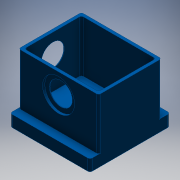
# Autodesk Inventor part: sampleChamber_singlePiece_filipeSample
Saved by Autodesk Inventor 2016 (Build 200138000, 138)
## iProperties
Created: 2016-04-10
Part Number: sampleChamber_singlePiece_filipeSample
Material: Generic
Document SubType Name: Modeling
Designer: sims01
Density: 1 g/cm^3
Appearance: Default
Author: sims01
Autodesk Inventor part; units mm, degrees
ref_plane "YZ Plane" through (0, 0, 0) normal (1, 0, 0) x (0, 1, 0)
ref_plane "XZ Plane" through (0, 0, 0) normal (0, 1, 0) x (-1, 0, 0)
ref_plane "XY Plane" through (0, 0, 0) normal (0, 0, 1) x (1, 0, 0)
sketch "Sketch1" plane through (0, 0, 0) normal (0, 0, 1) x (1, 0, 0)
  line L0 (-33, 35) -> (33, 35)
  line L1 (35, 33) -> (35, -33)
  line L2 (33, -35) -> (-33, -35)
  line L3 (-35, -33) -> (-35, 33)
  arc A0 (-35, -33) -> (-33, -35) centre (-33, -33) ccw
  arc A1 (-33, 35) -> (-35, 33) centre (-33, 33) ccw
  arc A2 (35, 33) -> (33, 35) centre (33, 33) ccw
  arc A3 (33, -35) -> (35, -33) centre (33, -33) ccw
  point P0 (0, 0)
  point P1 (-35, 35)
  point P2 (35, -35)
  point P3 (35, 35)
  point P4 (-35, -35)
  dimension "d0" = 70
  dimension "d1" = 35
  dimension "d2" = 70
  dimension "d3" = 35
  dimension "d85" = 2
  constraints: 8 end point, 8 point on circle, 8 point on line, 8 tangent, 4 centre point, 3 equal radius, 2 parallel, 1 horizontal, 1 perpendicular
  measures "d0" distance of point (35, -35) point (-35, -35)
  measures "d1" distance from line of point (0, 0) L1
  measures "d2" distance of point (-35, -35) point (-35, 35)
  measures "d3" distance from line of point (0, 0) L0
  measures "d85" radius of A0
extrude "Extrusion1" add sketch "Sketch1" along normal blind 10
sketch "Sketch3" plane through (0, 0, 10) normal (0, 0, 1) x (1, 0, 0)
  line L0 (-33, 27.5) -> (33, 27.5)
  line L1 (35, 25.5) -> (35, -25.5)
  line L2 (33, -27.5) -> (-33, -27.5)
  line L3 (-35, -25.5) -> (-35, 25.5)
  line L4 (-35, 33) -> (-35, -33) projected
  line L5 (-30.5, 25) -> (30.5, 25)
  line L6 (32.5, 23) -> (32.5, -23)
  line L7 (30.5, -25) -> (-30.5, -25)
  line L8 (-32.5, -23) -> (-32.5, 23)
  arc A0 (-35, -25.5) -> (-33, -27.5) centre (-33, -25.5) ccw
  arc A1 (-32.5, -23) -> (-30.5, -25) centre (-30.5, -23) ccw
  arc A2 (33, -27.5) -> (35, -25.5) centre (33, -25.5) ccw
  arc A3 (30.5, -25) -> (32.5, -23) centre (30.5, -23) ccw
  arc A4 (32.5, 23) -> (30.5, 25) centre (30.5, 23) ccw
  arc A5 (-30.5, 25) -> (-32.5, 23) centre (-30.5, 23) ccw
  arc A6 (-33, 27.5) -> (-35, 25.5) centre (-33, 25.5) ccw
  arc A7 (35, 25.5) -> (33, 27.5) centre (33, 25.5) ccw
  point P0 (0, 0)
  point P1 (-35, 27.5)
  point P2 (35, -27.5)
  point P3 (35, 27.5)
  point P4 (-35, -27.5)
  point P5 (-35, 35)
  point P6 (-35, -35)
  point P7 (-32.5, 25)
  point P8 (32.5, -25)
  point P9 (32.5, 25)
  point P10 (-32.5, -25)
  dimension "d17" = 70
  dimension "d18" = 55
  dimension "d19" = 27.5
  dimension "d20" = 2.5
  dimension "d21" = 2.5
  dimension "d22" = 2.5
  dimension "d23" = 2.5
  dimension "d86" = 2
  constraints: 16 end point, 16 point on circle, 16 point on line, 16 tangent, 8 centre point, 7 equal radius, 4 parallel, 2 horizontal, 2 perpendicular, 1 collinear
  measures "d17" distance of point (-35, 27.5) point (35, 27.5)
  measures "d18" distance of point (35, 27.5) point (35, -27.5)
  measures "d19" distance from line of L2 point (0, 0)
  measures "d20" distance between parallel lines of L5 L0
  measures "d21" distance between parallel lines of L1 L6
  measures "d22" distance between parallel lines of L2 L7
  measures "d23" distance between parallel lines of L3 L8
  measures "d86" radius of A0
extrude "Extrusion2" add sketch "Sketch3" along normal blind 45
sketch "Sketch9" plane through (-35, -27.5, 10) normal (0, -1, 0) x (1, 0, 0)
  circle A0 centre (35, 27.5) radius 14
  line L0 (0, 0) -> (0, 45) projected
  line L1 (2, 0) -> (68, 0) projected
  point P0 (35, -10)
  point P1 (70, 0)
  dimension "d60" = 28
  dimension "d61" = 35
  dimension "d62" = 27.5
  constraints: 1 centre point
  measures "d60" diameter of A0
  measures "d61" distance from line of L0 A0.centre
  measures "d62" distance from line of L1 A0.centre
extrude "Extrusion8" cut sketch "Sketch9" against normal blind 2
sketch "Sketch10" plane through (0, -25.5, 37.5) normal (0, -1, 0) x (1, 0, 0)
  circle A0 centre (0, 0) radius 10
  point P0 (0, -37.5)
  dimension "d65" = 20
  constraints: 1 centre point
  measures "d65" diameter of A0
extrude "Extrusion9" cut sketch "Sketch10" against normal blind 2
sketch "Sketch13" plane through (-35, -35, 0) normal (-1, 0, 0) x (0, 0, 1)
  circle A0 centre (37.5, 35) radius 14
  line L0 (0, 68) -> (0, 2) projected
  line L1 (10, 68) -> (10, 60.5) projected
  point P0 (0, 35)
  point P1 (0, 35)
  point P2 (0, 0)
  point P3 (0, 70)
  point P4 (10, 70)
  point P5 (10, 62.5)
  point P6 (10, 7.5)
  dimension "d76" = 28
  dimension "d82" = 27.5
  constraints: 1 centre point, 1 horizontal alignment, 1 midpoint
  measures "d76" diameter of A0
  measures "d82" distance from line of L1 A0.centre
extrude "Extrusion12" cut sketch "Sketch13" against normal blind 2
sketch "Sketch14" plane through (-33, 0, 37.5) normal (-1, 0, 0) x (0, 0, 1)
  circle A0 centre (0, 0) radius 10
  line L0 (-37.5, 33) -> (-37.5, -33) projected
  line L1 (-27.5, 33) -> (-27.5, 25.5) projected
  point P0 (-37.5, 0)
  point P1 (-37.5, 0)
  point P2 (-37.5, -35)
  point P3 (-37.5, 35)
  point P4 (-27.5, 35)
  point P5 (-27.5, 27.5)
  point P6 (-27.5, -27.5)
  dimension "d80" = 20
  dimension "d81" = 27.5
  constraints: 1 centre point, 1 horizontal alignment, 1 midpoint
  measures "d80" diameter of A0
  measures "d81" distance from line of L1 A0.centre
extrude "Extrusion13" cut sketch "Sketch14" against normal blind 2
equation "\"d1\" = 0.5 * d0"
equation "\"d3\" = 0.5 * d2"
equation "\"d19\" = 0.5 * d18"
equation "\"d21\" = d20"
body "Solid1"
